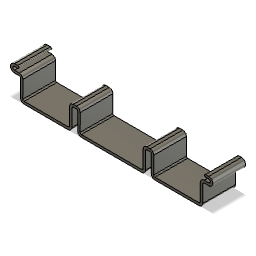
bracket c-thickness parameterized v3 (Autodesk Fusion 360 design; units mm, degrees)
Autodesk Fusion 360 part; units mm, degrees
note: some values were not read from the file. Set by a fixed rule: which sketch regions a step uses.
sketch "Sketch1" plane through (0, 0, 0) normal (0, 0, 1) x (1, 0, 0)
  line L0 (-0.5032, -3.4999) -> (2.3969, -3.5062) construction
  line L1 (3.8936, -5.0095) -> (3.8707, -15.5094) construction
  line L2 (5.3674, -17.0127) -> (32.3673, -17.0717) construction
  line L3 (33.8706, -15.575) -> (33.8935, -5.075) construction
  line L4 (35.3968, -3.5783) -> (37.3968, -3.5826) construction
  line L5 (38.8935, -5.0859) -> (38.8706, -15.5859) construction
  line L6 (40.3673, -17.0892) -> (58.8673, -17.1296) construction
  arc A0 (3.8707, -15.5094) -> (5.3674, -17.0127) centre (5.3707, -15.5127) ccw construction
  arc A1 (3.8936, -5.0095) -> (2.3969, -3.5062) centre (2.3936, -5.0062) ccw construction
  arc A2 (32.3673, -17.0717) -> (33.8706, -15.575) centre (32.3706, -15.5717) ccw construction
  arc A3 (35.3968, -3.5783) -> (33.8935, -5.075) centre (35.3935, -5.0783) ccw construction
  arc A4 (38.8935, -5.0859) -> (37.3968, -3.5826) centre (37.3935, -5.0826) ccw construction
  arc A5 (38.8706, -15.5859) -> (40.3673, -17.0892) centre (40.3706, -15.5892) ccw construction
  arc A6 (4.6436, -5.0111) -> (2.3985, -2.7562) centre (2.3936, -5.0062) ccw
  line L7 (-0.5049, -4.2499) -> (2.3952, -4.2562)
  line L8 (-0.5016, -2.7499) -> (2.3985, -2.7562)
  arc A7 (3.1436, -5.0078) -> (2.3952, -4.2562) centre (2.3936, -5.0062) ccw
  line L9 (3.1436, -5.0078) -> (3.1207, -15.5078)
  arc A8 (3.1207, -15.5078) -> (5.3658, -17.7627) centre (5.3707, -15.5127) ccw
  line L10 (5.3658, -17.7627) -> (32.3657, -17.8217)
  line L11 (4.6436, -5.0111) -> (4.6207, -15.5111)
  arc A9 (4.6207, -15.5111) -> (5.369, -16.2627) centre (5.3707, -15.5127) ccw
  line L12 (5.369, -16.2627) -> (32.369, -16.3217)
  arc A10 (32.369, -16.3217) -> (33.1206, -15.5733) centre (32.3706, -15.5717) ccw
  line L13 (33.1206, -15.5733) -> (33.1435, -5.0734)
  arc A11 (35.3984, -2.8283) -> (33.1435, -5.0734) centre (35.3935, -5.0783) ccw
  line L14 (35.3984, -2.8283) -> (37.3984, -2.8326)
  arc A12 (39.6435, -5.0876) -> (37.3984, -2.8326) centre (37.3935, -5.0826) ccw
  line L15 (39.6435, -5.0876) -> (39.6206, -15.5875)
  arc A13 (39.6206, -15.5875) -> (40.3689, -16.3392) centre (40.3706, -15.5892) ccw
  line L16 (40.3689, -16.3392) -> (58.8689, -16.3796)
  arc A14 (32.3657, -17.8217) -> (34.6206, -15.5766) centre (32.3706, -15.5717) ccw
  line L17 (34.6206, -15.5766) -> (34.6435, -5.0766)
  arc A15 (35.3952, -4.3283) -> (34.6435, -5.0766) centre (35.3935, -5.0783) ccw
  line L18 (35.3952, -4.3283) -> (37.3952, -4.3326)
  arc A16 (38.1435, -5.0843) -> (37.3952, -4.3326) centre (37.3935, -5.0826) ccw
  line L19 (38.1435, -5.0843) -> (38.1206, -15.5843)
  arc A17 (38.1206, -15.5843) -> (40.3657, -17.8392) centre (40.3706, -15.5892) ccw
  line L20 (40.3657, -17.8392) -> (58.8656, -17.8796)
  line L21 (58.8689, -16.3796) -> (58.8656, -17.8796)
  line L22 (-0.5016, -2.7499) -> (-0.4994, -1.7499) construction
  line L23 (-0.5049, -4.2499) -> (-0.4939, 0.7501) construction
  arc A18 (-0.4972, -0.7499) -> (-0.5016, -2.7499) centre (-0.4994, -1.7499) ccw
  arc A19 (-0.4939, 0.7501) -> (-0.5049, -4.2499) centre (-0.4994, -1.7499) ccw
  line L24 (-0.4972, -0.7499) -> (1.5028, -0.7542)
  line L25 (-0.4939, 0.7501) -> (1.5061, 0.7458)
  arc A20 (1.5028, -0.7542) -> (1.5061, 0.7458) centre (1.5044, -0.0042) ccw
  point P0 (3.8969, -3.5095)
  point P1 (3.8674, -17.0094)
  point P2 (33.8673, -17.075)
  point P3 (33.8968, -3.575)
  point P4 (38.8968, -3.5859)
  point P5 (38.8673, -17.0859)
  dimension "d34" = 30
  dimension "d35" = 13.5
  dimension "d36" = 5
  dimension "d37" = 13.5
  dimension "d38" = 20
  dimension "d39" = 1.5
  dimension "d40" = 1.5
  dimension "d41" = 1.5
  dimension "d42" = 1.5
  dimension "d43" = 1.5
  dimension "d44" = 1.5
  dimension "d49" = 0.75
  dimension "d52" = 0.75
  dimension "d53" = -0.75
  dimension "d54" = -0.75
  dimension "d55" = 0.75
  dimension "d56" = -0.75
  dimension "d57" = 0.75
  dimension "d58" = 0.75
  dimension "d59" = 1
  dimension "d60" = 2
  dimension "d62" = 5
  dimension "d67" = 2
  dimension "d68" = 2
  constraint perpendicular L0 L1
  constraint perpendicular L1 L2
  constraint perpendicular L2 L3
  constraint perpendicular L3 L4
  constraint perpendicular L4 L5
  constraint perpendicular L5 L6
  constraint coincident P1 L1
  constraint coincident P1 L2
  constraint tangent L1 A0
  constraint tangent L2 A0
  constraint coincident P0 L0
  constraint coincident P0 L1
  constraint tangent L0 A1
  constraint tangent L1 A1
  constraint coincident P2 L2
  constraint coincident P2 L3
  constraint tangent L2 A2
  constraint tangent L3 A2
  constraint coincident P3 L3
  constraint coincident P3 L4
  constraint tangent L3 A3
  constraint tangent L4 A3
  constraint coincident P4 L4
  constraint coincident P4 L5
  constraint tangent L4 A4
  constraint tangent L5 A4
  constraint coincident P5 L5
  constraint coincident P5 L6
  constraint tangent L5 A5
  constraint tangent L6 A5
  constraint perpendicular L20 L21
  constraint perpendicular L8 L22
  constraint coincident L22.end A18.centre
  constraint perpendicular L7 L23
  constraint coincident L23 A18.start
  constraint perpendicular L23 L24
  constraint perpendicular L23 L25
  constraint tangent L24 A20
  measures "d34" distance of P1 P2
  measures "d35" distance of P2 P3
  measures "d36" distance of P3 P4
  measures "d37" distance of P4 P5
  measures "d38" distance of P5 L6.end
  measures "d39" radius of A0
  measures "d40" radius of A1
  measures "d41" radius of A2
  measures "d42" radius of A3
  measures "d43" radius of A4
  measures "d44" radius of A5
  measures "d59" distance of L8.start L22.end
  measures "d60" diameter of A18
  measures "d62" distance of L7.start L23.end
  measures "d67" distance of A18.start L24.end
  measures "d68" distance of L23.end L25.end
extrude "Extrude1" add sketch "Sketch1" along normal blind 20
mirror "Mirror1" about plane through (58.8689, -16.3796, 0) normal (0.999998, -0.002184, 0) of bodies 1 merged
equation "h = 15 mm"
equation "d = 2 mm"
equation "t = 1.5 mm"
equation "i1 = 2 mm"
equation "i2 = 5 mm"
equation "i3 = 30 mm"
equation "w = 20 mm"
equation "i = 120 mm"
equation "d34 = i3"
equation "d35 = h - t"
equation "d36 = i2"
equation "d37 = h - t"
equation "d38 = i / 2 - 2 * i2 - i3"
equation "d39 = t"
equation "d40 = t"
equation "d41 = t"
equation "d42 = t"
equation "d43 = t"
equation "d44 = t"
equation "d49 = t / 2"
equation "d52 = t / 2"
equation "d53 = -t / 2"
equation "d54 = -t / 2"
equation "d55 = t / 2"
equation "d56 = -t / 2"
equation "d57 = t / 2"
equation "d58 = t / 2"
equation "d63 = w"
equation "d67 = i1"
equation "d68 = i1"
